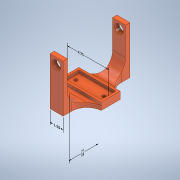
# Autodesk Inventor part: connectorToTubeBrackeCradle
Saved by Autodesk Inventor 2021.2 (Build 252289000, 289)
## iProperties
Created: 2020-07-23
Part Number: connectorToTubeBrackeCradle
Material: PBT Plastic
Document SubType Name: Modeling
Designer: robst
Density: 1.31 g/cm^3
Appearance: Smooth - Light Orange
Mass: 222.466 g
Surface Area: 338.142 cm^2
Volume: 169.821 cm^3
Author: robst
Autodesk Inventor part; units mm, degrees
ref_plane "YZ Plane" through (0, 0, 0) normal (1, 0, 0) x (0, 1, 0)
ref_plane "XZ Plane" through (0, 0, 0) normal (0, 1, 0) x (-1, 0, 0)
ref_plane "XY Plane" through (0, 0, 0) normal (0, 0, 1) x (1, 0, 0)
sketch "Sketch1" plane through (0, 0, 0) normal (0, 1, 0) x (-1, 0, 0)
  line L0 (53.975, 21.59) -> (-53.975, 21.59)
  line L1 (-53.975, 21.59) -> (-53.975, -21.59)
  line L2 (-53.975, -21.59) -> (53.975, -21.59)
  line L3 (53.975, -21.59) -> (53.975, 21.59)
  line L4 (53.975, 21.59) -> (-53.975, -21.59) construction
  line L5 (-53.975, 21.59) -> (53.975, -21.59) construction
  line L6 (60.325, 27.94) -> (-60.325, 27.94)
  line L7 (-60.325, 27.94) -> (-60.325, -27.94)
  line L8 (-60.325, -27.94) -> (60.325, -27.94)
  line L9 (60.325, -27.94) -> (60.325, 27.94)
  line L10 (60.325, 27.94) -> (-60.325, -27.94) construction
  line L11 (-60.325, 27.94) -> (60.325, -27.94) construction
  point P0 (0, 0)
  dimension "d0" = 43.18
  dimension "d1" = 107.95
  dimension "d2" = 6.35
  dimension "d3" = 6.35
  constraints: 24 end point, 4 midpoint, 4 parallel, 2 horizontal, 2 perpendicular
  measures "d0" distance of L0.end L1.end
  measures "d1" distance between parallel lines of L1 L3
  measures "d2" distance between parallel lines of L8 L2
  measures "d3" distance between parallel lines of L9 L3
extrude "Extrusion1" add sketch "Sketch1" against normal blind 12.065 contours L3 L2 L1 L0 | L9 L8 L7 L6
extrude "Extrusion2" add sketch "Sketch1" along normal blind 8.89
sketch "Sketch2" plane through (0, 0, 0) normal (0, 1, 0) x (1, 0, 0)
  line L0 (-53.975, 21.59) -> (-53.975, -21.59) construction
  line L1 (-53.975, 0) -> (53.975, 0) construction
  line L2 (53.975, -21.59) -> (53.975, 21.59) construction
  point P0 (0, 0)
  point P1 (-41.275, 0)
  point P2 (41.275, 0)
  dimension "d8" = 12.7
  dimension "d9" = 12.7
  constraints: 2 end point, 2 midpoint, 2 point on line
  measures "d8" distance from line of point (-41.275, 0) L0
  measures "d9" distance from line of point (41.275, 0) L2
hole "Hole1" at (-41.275, 0, 0) at (41.275, 0, 0) direction (0, -1, 0) diameter 5.1054 end through all counterbore diameter 10.16 counterbore depth 2.54 clearance for "Hex Machine Screw" size "#10" standard "Ansi Unified Screw Threads"
sketch "Sketch15" plane through (-60.325, -12.065, 27.94) normal (0, 0, 1) x (1, 0, 0)
  line L0 (0, 20.955) -> (120.65, 20.955) projected
  line L1 (120.65, 20.955) -> (120.65, 0) projected
  line L2 (120.65, 0) -> (0, 0) projected
  line L3 (0, 0) -> (0, 20.955) projected
  line L4 (0, 20.955) -> (120.65, 0) construction
  line L5 (0, 0) -> (120.65, 20.955) construction
  line L6 (41.275, 0) -> (79.375, 0)
  line L7 (79.375, 0) -> (79.375, 20.955)
  line L8 (79.375, 20.955) -> (41.275, 20.955)
  line L9 (41.275, 20.955) -> (41.275, 0)
  line L10 (41.275, 0) -> (79.375, 20.955) construction
  line L11 (79.375, 0) -> (41.275, 20.955) construction
  line L12 (114.3, 12.065) -> (6.35, 12.065) projected
  point P0 (60.325, 12.065)
  point P1 (60.325, 10.4775)
  point P2 (79.375, 12.065)
  point P3 (41.275, 12.065)
  point P4 (41.275, 0)
  point P5 (79.375, 0)
  dimension "d109" = 38.1
  constraints: 16 end point, 3 midpoint, 3 parallel, 1 collinear, 1 perpendicular
  measures "d109" distance between parallel lines of L7 L9
extrude "Extrusion10" add sketch "Sketch15" along normal blind 69.85 contours L12 L7 L2 L9
sketch "Sketch16" plane through (-19.05, 0, 27.94) normal (0, 1, 0) x (1, 0, 0)
  line L0 (0, -69.85) -> (38.1, -69.85) projected
  line L1 (38.1, 0) -> (38.1, -69.85) projected
  line L2 (0, -69.85) -> (38.1, -69.85)
  line L3 (38.1, -69.85) -> (38.1, -57.15)
  line L4 (38.1, -57.15) -> (0, -57.15)
  line L5 (0, -57.15) -> (0, -69.85)
  point P0 (19.05, 27.94)
  dimension "d103" = 12.7
  constraints: 8 end point, 2 parallel, 1 horizontal, 1 perpendicular, 1 point on line
  measures "d103" distance between parallel lines of L4 L0
extrude "Extrusion11" add sketch "Sketch16" along normal blind 127
sketch "Sketch17" plane through (-60.325, -12.065, 97.79) normal (0, 0, 1) x (1, 0, 0)
  line L0 (41.275, 139.065) -> (79.375, 139.065) construction
  line L1 (41.275, 0) -> (79.375, 0) construction
  line L2 (79.375, 139.065) -> (41.275, 139.065) construction
  line L3 (60.325, 139.065) -> (60.325, 0) construction
  circle A0 centre (60.325, 120.015) radius 12.7
  point P0 (60.325, 12.065)
  dimension "d113" = 25.4
  dimension "d114" = 19.05
  constraints: 2 end point, 2 midpoint, 1 centre point, 1 point on line
  measures "d113" diameter of A0
  measures "d114" distance from line of A0.centre L0
extrude "Extrusion12" cut sketch "Sketch17" against normal through all
mirror "Mirror8" about plane through (0, 0, 0) normal (0, 0, 1) of "Extrusion11", "Extrusion12", "Extrusion10"
fillet "Fillet1" radius 44.45 2 edges at (0, 0, -85.09) (0, 0, 85.09)
fillet "Fillet2" radius 44.45 4 edges at (19.05, -6.0325, -27.94) (19.05, -6.0325, 27.94) (-19.05, -6.0325, -27.94) (-19.05, -6.0325, 27.94)
equation "\"d0\" = innerWidth"
equation "\"d1\" = innerLength"
equation "\"d2\" = wallThickness"
equation "\"d3\" = wallThickness"
equation "\"d4\" = bottomThickness"
equation "\"d6\" = innerDepth"
equation "\"d8\" = holeCenterFromInnerWall"
equation "\"d9\" = holeCenterFromInnerWall"
equation "\"innerWidth\" = 43.18"
equation "\"innerLength\" = 107.95"
equation "\"innerDepth\" = 8.89"
equation "\"wallThickness\" = 6.35"
equation "\"postDiameter\" = 9.525"
equation "\"holeCenterFromInnerWall\" = 12.7"
equation "\"bottomThickness\" = 12.065"
equation "\"d17\" = postDiameter"
equation "\"exteriorWidth\" = innerWidth + 2 * wallThickness"
equation "\"exteriorLength\" = innerLength + 2 * wallThickness"
equation "\"exteriorHeight\" = innerDepth + bottomThickness"
equation "\"d24\" = postDiameter"
equation "\"lowerPostWidth\" = exteriorWidth"
equation "\"lowerPostLength\" = 50.8"
equation "\"lowerPostCenterX\" = 0.5 * exteriorLength"
equation "\"lowerPostHeight\" = 19.05"
equation "\"lowerPostCenterY\" = postDiameter"
equation "\"setScrewCenters\" = 0.333333 * exteriorWidth"
equation "\"hexSize\" = 12.7"
body "Solid1"
